Autodesk Fusion 360 part; units mm, degrees
(part 3 of 9)
  line L659 (-69.109, 106.2894) -> (-73.4391, 108.7894)
  line L660 (-63.2789, 108.7894) -> (-67.609, 106.2894)
  line L661 (-67.609, 106.2894) -> (-67.609, 101.2894)
  line L662 (-67.609, 101.2894) -> (-63.2789, 98.7894)
  line L663 (-63.2789, 98.7894) -> (-58.9487, 101.2894)
  line L664 (-58.9487, 101.2894) -> (-58.9487, 106.2894)
  line L665 (-58.9487, 106.2894) -> (-63.2789, 108.7894)
  line L666 (-53.1186, 108.7894) -> (-57.4487, 106.2894)
  line L667 (-57.4487, 106.2894) -> (-57.4487, 101.2894)
  line L668 (-57.4487, 101.2894) -> (-53.1186, 98.7894)
  line L669 (-53.1186, 98.7894) -> (-48.7885, 101.2894)
  line L670 (-48.7885, 101.2894) -> (-48.7885, 106.2894)
  line L671 (-48.7885, 106.2894) -> (-53.1186, 108.7894)
  line L672 (-42.9584, 108.7894) -> (-47.2885, 106.2894)
  line L673 (-47.2885, 106.2894) -> (-47.2885, 101.2894)
  line L674 (-47.2885, 101.2894) -> (-42.9584, 98.7894)
  line L675 (-42.9584, 98.7894) -> (-38.6282, 101.2894)
  line L676 (-38.6282, 101.2894) -> (-38.6282, 106.2894)
  line L677 (-38.6282, 106.2894) -> (-42.9584, 108.7894)
  line L678 (-32.7981, 108.7894) -> (-37.1282, 106.2894)
  line L679 (-37.1282, 106.2894) -> (-37.1282, 101.2894)
  line L680 (-37.1282, 101.2894) -> (-32.7981, 98.7894)
  line L681 (-32.7981, 98.7894) -> (-28.468, 101.2894)
  line L682 (-28.468, 101.2894) -> (-28.468, 106.2894)
  line L683 (-28.468, 106.2894) -> (-32.7981, 108.7894)
  line L684 (-22.6378, 108.7894) -> (-26.968, 106.2894)
  line L685 (-26.968, 106.2894) -> (-26.968, 101.2894)
  line L686 (-26.968, 101.2894) -> (-22.6378, 98.7894)
  line L687 (-22.6378, 98.7894) -> (-18.3077, 101.2894)
  line L688 (-18.3077, 101.2894) -> (-18.3077, 106.2894)
  line L689 (-18.3077, 106.2894) -> (-22.6378, 108.7894)
  line L690 (-12.4776, 108.7894) -> (-16.8077, 106.2894)
  line L691 (-16.8077, 106.2894) -> (-16.8077, 101.2894)
  line L692 (-16.8077, 101.2894) -> (-12.4776, 98.7894)
  line L693 (-12.4776, 98.7894) -> (-8.1475, 101.2894)
  line L694 (-8.1475, 101.2894) -> (-8.1475, 106.2894)
  line L695 (-8.1475, 106.2894) -> (-12.4776, 108.7894)
  line L696 (-109, 117.5885) -> (-113.3301, 115.0885)
  line L697 (-113.3301, 115.0885) -> (-113.3301, 110.0885)
  line L698 (-113.3301, 110.0885) -> (-109, 107.5885)
  line L699 (-109, 107.5885) -> (-104.6699, 110.0885)
  line L700 (-104.6699, 110.0885) -> (-104.6699, 115.0885)
  line L701 (-104.6699, 115.0885) -> (-109, 117.5885)
  line L702 (-98.8397, 117.5885) -> (-103.1699, 115.0885)
  line L703 (-103.1699, 115.0885) -> (-103.1699, 110.0885)
  line L704 (-103.1699, 110.0885) -> (-98.8397, 107.5885)
  line L705 (-98.8397, 107.5885) -> (-94.5096, 110.0885)
  line L706 (-94.5096, 110.0885) -> (-94.5096, 115.0885)
  line L707 (-94.5096, 115.0885) -> (-98.8397, 117.5885)
  line L708 (-88.6795, 117.5885) -> (-93.0096, 115.0885)
  line L709 (-93.0096, 115.0885) -> (-93.0096, 110.0885)
  line L710 (-93.0096, 110.0885) -> (-88.6795, 107.5885)
  line L711 (-88.6795, 107.5885) -> (-84.3494, 110.0885)
  line L712 (-84.3494, 110.0885) -> (-84.3494, 115.0885)
  line L713 (-84.3494, 115.0885) -> (-88.6795, 117.5885)
  line L714 (-78.5192, 117.5885) -> (-82.8494, 115.0885)
  line L715 (-82.8494, 115.0885) -> (-82.8494, 110.0885)
  line L716 (-82.8494, 110.0885) -> (-78.5192, 107.5885)
  line L717 (-78.5192, 107.5885) -> (-74.1891, 110.0885)
  line L718 (-74.1891, 110.0885) -> (-74.1891, 115.0885)
  line L719 (-74.1891, 115.0885) -> (-78.5192, 117.5885)
  line L720 (-68.359, 117.5885) -> (-72.6891, 115.0885)
  line L721 (-72.6891, 115.0885) -> (-72.6891, 110.0885)
  line L722 (-72.6891, 110.0885) -> (-68.359, 107.5885)
  line L723 (-68.359, 107.5885) -> (-64.0289, 110.0885)
  line L724 (-64.0289, 110.0885) -> (-64.0289, 115.0885)
  line L725 (-64.0289, 115.0885) -> (-68.359, 117.5885)
  line L726 (-58.1987, 117.5885) -> (-62.5289, 115.0885)
  line L727 (-62.5289, 115.0885) -> (-62.5289, 110.0885)
  line L728 (-62.5289, 110.0885) -> (-58.1987, 107.5885)
  line L729 (-58.1987, 107.5885) -> (-53.8686, 110.0885)
  line L730 (-53.8686, 110.0885) -> (-53.8686, 115.0885)
  line L731 (-53.8686, 115.0885) -> (-58.1987, 117.5885)
  line L732 (-48.0385, 117.5885) -> (-52.3686, 115.0885)
  line L733 (-52.3686, 115.0885) -> (-52.3686, 110.0885)
  line L734 (-52.3686, 110.0885) -> (-48.0385, 107.5885)
  line L735 (-48.0385, 107.5885) -> (-43.7084, 110.0885)
  line L736 (-43.7084, 110.0885) -> (-43.7084, 115.0885)
  line L737 (-43.7084, 115.0885) -> (-48.0385, 117.5885)
  line L738 (-37.8782, 117.5885) -> (-42.2084, 115.0885)
  line L739 (-42.2084, 115.0885) -> (-42.2084, 110.0885)
  line L740 (-42.2084, 110.0885) -> (-37.8782, 107.5885)
  line L741 (-37.8782, 107.5885) -> (-33.5481, 110.0885)
  line L742 (-33.5481, 110.0885) -> (-33.5481, 115.0885)
  line L743 (-33.5481, 115.0885) -> (-37.8782, 117.5885)
  line L744 (-27.718, 117.5885) -> (-32.0481, 115.0885)
  line L745 (-32.0481, 115.0885) -> (-32.0481, 110.0885)
  line L746 (-32.0481, 110.0885) -> (-27.718, 107.5885)
  line L747 (-27.718, 107.5885) -> (-23.3878, 110.0885)
  line L748 (-23.3878, 110.0885) -> (-23.3878, 115.0885)
  line L749 (-23.3878, 115.0885) -> (-27.718, 117.5885)
  line L750 (-17.5577, 117.5885) -> (-21.8878, 115.0885)
  line L751 (-21.8878, 115.0885) -> (-21.8878, 110.0885)
  line L752 (-21.8878, 110.0885) -> (-17.5577, 107.5885)
  line L753 (-17.5577, 107.5885) -> (-13.2276, 110.0885)
  line L754 (-13.2276, 110.0885) -> (-13.2276, 115.0885)
  line L755 (-13.2276, 115.0885) -> (-17.5577, 117.5885)
  line L756 (-7.3975, 117.5885) -> (-11.7276, 115.0885)
  line L757 (-11.7276, 115.0885) -> (-11.7276, 110.0885)
  line L758 (-11.7276, 110.0885) -> (-7.3975, 107.5885)
  line L759 (-7.3975, 107.5885) -> (-3.0673, 110.0885)
  line L760 (-3.0673, 110.0885) -> (-3.0673, 115.0885)
  line L761 (-3.0673, 115.0885) -> (-7.3975, 117.5885)
  line L762 (-103.9199, 126.3875) -> (-108.25, 123.8875)
  line L763 (-108.25, 123.8875) -> (-108.25, 118.8875)
  line L764 (-108.25, 118.8875) -> (-103.9199, 116.3875)
  line L765 (-103.9199, 116.3875) -> (-99.5897, 118.8875)
  line L766 (-99.5897, 118.8875) -> (-99.5897, 123.8875)
  line L767 (-99.5897, 123.8875) -> (-103.9199, 126.3875)
  line L768 (-93.7596, 126.3875) -> (-98.0897, 123.8875)
  line L769 (-98.0897, 123.8875) -> (-98.0897, 118.8875)
  line L770 (-98.0897, 118.8875) -> (-93.7596, 116.3875)
  line L771 (-93.7596, 116.3875) -> (-89.4295, 118.8875)
  line L772 (-89.4295, 118.8875) -> (-89.4295, 123.8875)
  line L773 (-89.4295, 123.8875) -> (-93.7596, 126.3875)
  line L774 (-83.5994, 126.3875) -> (-87.9295, 123.8875)
  line L775 (-87.9295, 123.8875) -> (-87.9295, 118.8875)
  line L776 (-87.9295, 118.8875) -> (-83.5994, 116.3875)
  line L777 (-83.5994, 116.3875) -> (-79.2692, 118.8875)
  line L778 (-79.2692, 118.8875) -> (-79.2692, 123.8875)
  line L779 (-79.2692, 123.8875) -> (-83.5994, 126.3875)
  line L780 (-73.4391, 126.3875) -> (-77.7692, 123.8875)
  line L781 (-77.7692, 123.8875) -> (-77.7692, 118.8875)
  line L782 (-77.7692, 118.8875) -> (-73.4391, 116.3875)
  line L783 (-73.4391, 116.3875) -> (-69.109, 118.8875)
  line L784 (-69.109, 118.8875) -> (-69.109, 123.8875)
  line L785 (-69.109, 123.8875) -> (-73.4391, 126.3875)
  line L786 (-63.2789, 126.3875) -> (-67.609, 123.8875)
  line L787 (-67.609, 123.8875) -> (-67.609, 118.8875)
  line L788 (-67.609, 118.8875) -> (-63.2789, 116.3875)
  line L789 (-63.2789, 116.3875) -> (-58.9487, 118.8875)
  line L790 (-58.9487, 118.8875) -> (-58.9487, 123.8875)
  line L791 (-58.9487, 123.8875) -> (-63.2789, 126.3875)
  line L792 (-53.1186, 126.3875) -> (-57.4487, 123.8875)
  line L793 (-57.4487, 123.8875) -> (-57.4487, 118.8875)
  line L794 (-57.4487, 118.8875) -> (-53.1186, 116.3875)
  line L795 (-53.1186, 116.3875) -> (-48.7885, 118.8875)
  line L796 (-48.7885, 118.8875) -> (-48.7885, 123.8875)
  line L797 (-48.7885, 123.8875) -> (-53.1186, 126.3875)
  line L798 (-42.9584, 126.3875) -> (-47.2885, 123.8875)
  line L799 (-47.2885, 123.8875) -> (-47.2885, 118.8875)
  line L800 (-47.2885, 118.8875) -> (-42.9584, 116.3875)
  line L801 (-42.9584, 116.3875) -> (-38.6282, 118.8875)
  line L802 (-38.6282, 118.8875) -> (-38.6282, 123.8875)
  line L803 (-38.6282, 123.8875) -> (-42.9584, 126.3875)
  line L804 (-32.7981, 126.3875) -> (-37.1282, 123.8875)
  line L805 (-37.1282, 123.8875) -> (-37.1282, 118.8875)
  line L806 (-37.1282, 118.8875) -> (-32.7981, 116.3875)
  line L807 (-32.7981, 116.3875) -> (-28.468, 118.8875)
  line L808 (-28.468, 118.8875) -> (-28.468, 123.8875)
  line L809 (-28.468, 123.8875) -> (-32.7981, 126.3875)
  line L810 (-22.6378, 126.3875) -> (-26.968, 123.8875)
  line L811 (-26.968, 123.8875) -> (-26.968, 118.8875)
  line L812 (-26.968, 118.8875) -> (-22.6378, 116.3875)
  line L813 (-22.6378, 116.3875) -> (-18.3077, 118.8875)
  line L814 (-18.3077, 118.8875) -> (-18.3077, 123.8875)
  line L815 (-18.3077, 123.8875) -> (-22.6378, 126.3875)
  line L816 (-12.4776, 126.3875) -> (-16.8077, 123.8875)
  line L817 (-16.8077, 123.8875) -> (-16.8077, 118.8875)
  line L818 (-16.8077, 118.8875) -> (-12.4776, 116.3875)
  line L819 (-12.4776, 116.3875) -> (-8.1475, 118.8875)
  line L820 (-8.1475, 118.8875) -> (-8.1475, 123.8875)
  line L821 (-8.1475, 123.8875) -> (-12.4776, 126.3875)
  line L822 (-109, 135.1865) -> (-113.3301, 132.6865)
  line L823 (-113.3301, 132.6865) -> (-113.3301, 127.6865)
  line L824 (-113.3301, 127.6865) -> (-109, 125.1865)
  line L825 (-109, 125.1865) -> (-104.6699, 127.6865)
  line L826 (-104.6699, 127.6865) -> (-104.6699, 132.6865)
  line L827 (-104.6699, 132.6865) -> (-109, 135.1865)
  line L828 (-98.8397, 135.1865) -> (-103.1699, 132.6865)
  line L829 (-103.1699, 132.6865) -> (-103.1699, 127.6865)
  line L830 (-103.1699, 127.6865) -> (-98.8397, 125.1865)
  line L831 (-98.8397, 125.1865) -> (-94.5096, 127.6865)
  line L832 (-94.5096, 127.6865) -> (-94.5096, 132.6865)
  line L833 (-94.5096, 132.6865) -> (-98.8397, 135.1865)
  line L834 (-88.6795, 135.1865) -> (-93.0096, 132.6865)
  line L835 (-93.0096, 132.6865) -> (-93.0096, 127.6865)
  line L836 (-93.0096, 127.6865) -> (-88.6795, 125.1865)
  line L837 (-88.6795, 125.1865) -> (-84.3494, 127.6865)
  line L838 (-84.3494, 127.6865) -> (-84.3494, 132.6865)
  line L839 (-84.3494, 132.6865) -> (-88.6795, 135.1865)
  line L840 (-78.5192, 135.1865) -> (-82.8494, 132.6865)
  line L841 (-82.8494, 132.6865) -> (-82.8494, 127.6865)
  line L842 (-82.8494, 127.6865) -> (-78.5192, 125.1865)
  line L843 (-78.5192, 125.1865) -> (-74.1891, 127.6865)
  line L844 (-74.1891, 127.6865) -> (-74.1891, 132.6865)
  line L845 (-74.1891, 132.6865) -> (-78.5192, 135.1865)
  line L846 (-68.359, 135.1865) -> (-72.6891, 132.6865)
  line L847 (-72.6891, 132.6865) -> (-72.6891, 127.6865)
  line L848 (-72.6891, 127.6865) -> (-68.359, 125.1865)
  line L849 (-68.359, 125.1865) -> (-64.0289, 127.6865)
  line L850 (-64.0289, 127.6865) -> (-64.0289, 132.6865)
  line L851 (-64.0289, 132.6865) -> (-68.359, 135.1865)
  line L852 (-58.1987, 135.1865) -> (-62.5289, 132.6865)
  line L853 (-62.5289, 132.6865) -> (-62.5289, 127.6865)
  line L854 (-62.5289, 127.6865) -> (-58.1987, 125.1865)
  line L855 (-58.1987, 125.1865) -> (-53.8686, 127.6865)
  line L856 (-53.8686, 127.6865) -> (-53.8686, 132.6865)
  line L857 (-53.8686, 132.6865) -> (-58.1987, 135.1865)
  line L858 (-48.0385, 135.1865) -> (-52.3686, 132.6865)
  line L859 (-52.3686, 132.6865) -> (-52.3686, 127.6865)
  line L860 (-52.3686, 127.6865) -> (-48.0385, 125.1865)
  line L861 (-48.0385, 125.1865) -> (-43.7084, 127.6865)
  line L862 (-43.7084, 127.6865) -> (-43.7084, 132.6865)
  line L863 (-43.7084, 132.6865) -> (-48.0385, 135.1865)
  line L864 (-37.8782, 135.1865) -> (-42.2084, 132.6865)
  line L865 (-42.2084, 132.6865) -> (-42.2084, 127.6865)
  line L866 (-42.2084, 127.6865) -> (-37.8782, 125.1865)
  line L867 (-37.8782, 125.1865) -> (-33.5481, 127.6865)
  line L868 (-33.5481, 127.6865) -> (-33.5481, 132.6865)
  line L869 (-33.5481, 132.6865) -> (-37.8782, 135.1865)
  line L870 (-27.718, 135.1865) -> (-32.0481, 132.6865)
  line L871 (-32.0481, 132.6865) -> (-32.0481, 127.6865)
  line L872 (-32.0481, 127.6865) -> (-27.718, 125.1865)
  line L873 (-27.718, 125.1865) -> (-23.3878, 127.6865)
  line L874 (-23.3878, 127.6865) -> (-23.3878, 132.6865)
  line L875 (-23.3878, 132.6865) -> (-27.718, 135.1865)
  line L876 (-17.5577, 135.1865) -> (-21.8878, 132.6865)
  line L877 (-21.8878, 132.6865) -> (-21.8878, 127.6865)
  line L878 (-21.8878, 127.6865) -> (-17.5577, 125.1865)
  line L879 (-17.5577, 125.1865) -> (-13.2276, 127.6865)
  line L880 (-13.2276, 127.6865) -> (-13.2276, 132.6865)
  line L881 (-13.2276, 132.6865) -> (-17.5577, 135.1865)
  line L882 (-7.3975, 135.1865) -> (-11.7276, 132.6865)
  line L883 (-11.7276, 132.6865) -> (-11.7276, 127.6865)
  line L884 (-11.7276, 127.6865) -> (-7.3975, 125.1865)
  line L885 (-7.3975, 125.1865) -> (-3.0673, 127.6865)
  line L886 (-3.0673, 127.6865) -> (-3.0673, 132.6865)
  line L887 (-3.0673, 132.6865) -> (-7.3975, 135.1865)
  line L888 (-103.9199, 143.9856) -> (-108.25, 141.4856)
  line L889 (-108.25, 141.4856) -> (-108.25, 136.4856)
  line L890 (-108.25, 136.4856) -> (-103.9199, 133.9856)
  line L891 (-103.9199, 133.9856) -> (-99.5897, 136.4856)
  line L892 (-99.5897, 136.4856) -> (-99.5897, 141.4856)
  line L893 (-99.5897, 141.4856) -> (-103.9199, 143.9856)
  line L894 (-93.7596, 143.9856) -> (-98.0897, 141.4856)
  line L895 (-98.0897, 141.4856) -> (-98.0897, 136.4856)
  line L896 (-98.0897, 136.4856) -> (-93.7596, 133.9856)
  line L897 (-93.7596, 133.9856) -> (-89.4295, 136.4856)
  line L898 (-89.4295, 136.4856) -> (-89.4295, 141.4856)
  line L899 (-89.4295, 141.4856) -> (-93.7596, 143.9856)
  line L900 (-83.5994, 143.9856) -> (-87.9295, 141.4856)
  line L901 (-87.9295, 141.4856) -> (-87.9295, 136.4856)
  line L902 (-87.9295, 136.4856) -> (-83.5994, 133.9856)
  line L903 (-83.5994, 133.9856) -> (-79.2692, 136.4856)
  line L904 (-79.2692, 136.4856) -> (-79.2692, 141.4856)
  line L905 (-79.2692, 141.4856) -> (-83.5994, 143.9856)
  line L906 (-73.4391, 143.9856) -> (-77.7692, 141.4856)
  line L907 (-77.7692, 141.4856) -> (-77.7692, 136.4856)
  line L908 (-77.7692, 136.4856) -> (-73.4391, 133.9856)
  line L909 (-73.4391, 133.9856) -> (-69.109, 136.4856)
  line L910 (-69.109, 136.4856) -> (-69.109, 141.4856)
  line L911 (-69.109, 141.4856) -> (-73.4391, 143.9856)
  line L912 (-63.2789, 143.9856) -> (-67.609, 141.4856)
  line L913 (-67.609, 141.4856) -> (-67.609, 136.4856)
  line L914 (-67.609, 136.4856) -> (-63.2789, 133.9856)
  line L915 (-63.2789, 133.9856) -> (-58.9487, 136.4856)
  line L916 (-58.9487, 136.4856) -> (-58.9487, 141.4856)
  line L917 (-58.9487, 141.4856) -> (-63.2789, 143.9856)
  line L918 (-53.1186, 143.9856) -> (-57.4487, 141.4856)
  line L919 (-57.4487, 141.4856) -> (-57.4487, 136.4856)
  line L920 (-57.4487, 136.4856) -> (-53.1186, 133.9856)
  line L921 (-53.1186, 133.9856) -> (-48.7885, 136.4856)
  line L922 (-48.7885, 136.4856) -> (-48.7885, 141.4856)
  line L923 (-48.7885, 141.4856) -> (-53.1186, 143.9856)
  line L924 (-42.9584, 143.9856) -> (-47.2885, 141.4856)
  line L925 (-47.2885, 141.4856) -> (-47.2885, 136.4856)
  line L926 (-47.2885, 136.4856) -> (-42.9584, 133.9856)
  line L927 (-42.9584, 133.9856) -> (-38.6282, 136.4856)
  line L928 (-38.6282, 136.4856) -> (-38.6282, 141.4856)
  line L929 (-38.6282, 141.4856) -> (-42.9584, 143.9856)
  line L930 (-32.7981, 143.9856) -> (-37.1282, 141.4856)
  line L931 (-37.1282, 141.4856) -> (-37.1282, 136.4856)
  line L932 (-37.1282, 136.4856) -> (-32.7981, 133.9856)
  line L933 (-32.7981, 133.9856) -> (-28.468, 136.4856)
  line L934 (-28.468, 136.4856) -> (-28.468, 141.4856)
  line L935 (-28.468, 141.4856) -> (-32.7981, 143.9856)
  line L936 (-22.6378, 143.9856) -> (-26.968, 141.4856)
  line L937 (-26.968, 141.4856) -> (-26.968, 136.4856)
  line L938 (-26.968, 136.4856) -> (-22.6378, 133.9856)
  line L939 (-22.6378, 133.9856) -> (-18.3077, 136.4856)
  line L940 (-18.3077, 136.4856) -> (-18.3077, 141.4856)
  line L941 (-18.3077, 141.4856) -> (-22.6378, 143.9856)
  line L942 (-12.4776, 143.9856) -> (-16.8077, 141.4856)
  line L943 (-16.8077, 141.4856) -> (-16.8077, 136.4856)
  line L944 (-16.8077, 136.4856) -> (-12.4776, 133.9856)
  line L945 (-12.4776, 133.9856) -> (-8.1475, 136.4856)
  line L946 (-8.1475, 136.4856) -> (-8.1475, 141.4856)
  line L947 (-8.1475, 141.4856) -> (-12.4776, 143.9856)
  line L948 (-109, 152.7846) -> (-113.3301, 150.2846)
  line L949 (-113.3301, 150.2846) -> (-113.3301, 145.2846)
  line L950 (-113.3301, 145.2846) -> (-109, 142.7846)
  line L951 (-109, 142.7846) -> (-104.6699, 145.2846)
  line L952 (-104.6699, 145.2846) -> (-104.6699, 150.2846)
  line L953 (-104.6699, 150.2846) -> (-109, 152.7846)
  line L954 (-98.8397, 152.7846) -> (-103.1699, 150.2846)
  line L955 (-103.1699, 150.2846) -> (-103.1699, 145.2846)
  line L956 (-103.1699, 145.2846) -> (-98.8397, 142.7846)
  line L957 (-98.8397, 142.7846) -> (-94.5096, 145.2846)
  line L958 (-94.5096, 145.2846) -> (-94.5096, 150.2846)
  line L959 (-94.5096, 150.2846) -> (-98.8397, 152.7846)
  line L960 (-88.6795, 152.7846) -> (-93.0096, 150.2846)
  line L961 (-93.0096, 150.2846) -> (-93.0096, 145.2846)
  line L962 (-93.0096, 145.2846) -> (-88.6795, 142.7846)
  line L963 (-88.6795, 142.7846) -> (-84.3494, 145.2846)
  line L964 (-84.3494, 145.2846) -> (-84.3494, 150.2846)
  line L965 (-84.3494, 150.2846) -> (-88.6795, 152.7846)
  line L966 (-78.5192, 152.7846) -> (-82.8494, 150.2846)
  line L967 (-82.8494, 150.2846) -> (-82.8494, 145.2846)
  line L968 (-82.8494, 145.2846) -> (-78.5192, 142.7846)
  line L969 (-78.5192, 142.7846) -> (-74.1891, 145.2846)
  line L970 (-74.1891, 145.2846) -> (-74.1891, 150.2846)
  line L971 (-74.1891, 150.2846) -> (-78.5192, 152.7846)
  line L972 (-68.359, 152.7846) -> (-72.6891, 150.2846)
  line L973 (-72.6891, 150.2846) -> (-72.6891, 145.2846)
  line L974 (-72.6891, 145.2846) -> (-68.359, 142.7846)
  line L975 (-68.359, 142.7846) -> (-64.0289, 145.2846)
  line L976 (-64.0289, 145.2846) -> (-64.0289, 150.2846)
  line L977 (-64.0289, 150.2846) -> (-68.359, 152.7846)
  line L978 (-58.1987, 152.7846) -> (-62.5289, 150.2846)
  line L979 (-62.5289, 150.2846) -> (-62.5289, 145.2846)
  line L980 (-62.5289, 145.2846) -> (-58.1987, 142.7846)
  line L981 (-58.1987, 142.7846) -> (-53.8686, 145.2846)
  line L982 (-53.8686, 145.2846) -> (-53.8686, 150.2846)
  line L983 (-53.8686, 150.2846) -> (-58.1987, 152.7846)
  line L984 (-48.0385, 152.7846) -> (-52.3686, 150.2846)
  line L985 (-52.3686, 150.2846) -> (-52.3686, 145.2846)
  line L986 (-52.3686, 145.2846) -> (-48.0385, 142.7846)
  line L987 (-48.0385, 142.7846) -> (-43.7084, 145.2846)
  line L988 (-43.7084, 145.2846) -> (-43.7084, 150.2846)
  line L989 (-43.7084, 150.2846) -> (-48.0385, 152.7846)
  line L990 (-37.8782, 152.7846) -> (-42.2084, 150.2846)
  line L991 (-42.2084, 150.2846) -> (-42.2084, 145.2846)
  line L992 (-42.2084, 145.2846) -> (-37.8782, 142.7846)
  line L993 (-37.8782, 142.7846) -> (-33.5481, 145.2846)
  line L994 (-33.5481, 145.2846) -> (-33.5481, 150.2846)
  line L995 (-33.5481, 150.2846) -> (-37.8782, 152.7846)
  line L996 (-27.718, 152.7846) -> (-32.0481, 150.2846)
  line L997 (-32.0481, 150.2846) -> (-32.0481, 145.2846)
  line L998 (-32.0481, 145.2846) -> (-27.718, 142.7846)
  line L999 (-27.718, 142.7846) -> (-23.3878, 145.2846)
  line L1000 (-23.3878, 145.2846) -> (-23.3878, 150.2846)
  line L1001 (-23.3878, 150.2846) -> (-27.718, 152.7846)
  line L1002 (-17.5577, 152.7846) -> (-21.8878, 150.2846)
  line L1003 (-21.8878, 150.2846) -> (-21.8878, 145.2846)
  line L1004 (-21.8878, 145.2846) -> (-17.5577, 142.7846)
  line L1005 (-17.5577, 142.7846) -> (-13.2276, 145.2846)
  line L1006 (-13.2276, 145.2846) -> (-13.2276, 150.2846)
  line L1007 (-13.2276, 150.2846) -> (-17.5577, 152.7846)
  line L1008 (-7.3975, 152.7846) -> (-11.7276, 150.2846)
  line L1009 (-11.7276, 150.2846) -> (-11.7276, 145.2846)
  line L1010 (-11.7276, 145.2846) -> (-7.3975, 142.7846)
  line L1011 (-7.3975, 142.7846) -> (-3.0673, 145.2846)
  line L1012 (-3.0673, 145.2846) -> (-3.0673, 150.2846)
  line L1013 (-3.0673, 150.2846) -> (-7.3975, 152.7846)
extrude "拉伸22" cut sketch "草图21" against normal blind 5 contours L6 L7 L8 L9 L10 L11 | L12 L13 L14 L15 L16 L17 | L18 L19 L20 L21 L22 L23 | L24 L25 L26 L27 L28 L29 | L30 L31 L32 L33 L34 L35 | L36 L37 L38 L39 L40 L41 | L42 L43 L44 L45 L46 L47 | L48 L49 L50 L51 L52 L53 | L54 L55 L56 L57 L58 L59 | L60 L61 L62 L63 L64 L65 | L66 L67 L68 L69 L70 L71 | L72 L73 L74 L75 L76 L77 | L78 L79 L80 L81 L82 L83 | L84 L85 L86 L87 L88 L89 | L90 L91 L92 L93 L94 L95 | L96 L97 L98 L99 L100 L101 | L102 L103 L104 L105 L106 L107 | L108 L109 L110 L111 L112 L113 | L114 L115 L116 L117 L118 L119 | L120 L121 L122 L123 L124 L125 | L126 L127 L128 L129 L130 L131 | L132 L133 L134 L135 L136 L137 | L138 L139 L140 L141 L142 L143 | L144 L145 L146 L147 L148 L149 | L150 L151 L152 L153 L154 L155 | L156 L157 L158 L159 L160 L161 | L162 L163 L164 L165 L166 L167 | L168 L169 L170 L171 L172 L173 | L174 L175 L176 L177 L178 L179 | L180 L181 L182 L183 L184 L185 | L186 L187 L188 L189 L190 L191 | L192 L193 L194 L195 L196 L197 | L198 L199 L200 L201 L202 L203 | L204 L205 L206 L207 L208 L209 | L210 L211 L212 L213 L214 L215 | L216 L217 L218 L219 L220 L221 | L222 L223 L224 L225 L226 L227 | L228 L229 L230 L231 L232 L233 | L234 L235 L236 L237 L238 L239 | L240 L241 L242 L243 L244 L245 | L246 L247 L248 L249 L250 L251 | L252 L253 L254 L255 L256 L257 | L258 L259 L260 L261 L262 L263 | L264 L265 L266 L267 L268 L269 | L270 L271 L272 L273 L274 L275 | L276 L277 L278 L279 L280 L281 | L282 L283 L284 L285 L286 L287 | L288 L289 L290 L291 L292 L293 | L294 L295 L296 L297 L298 L299 | L300 L301 L302 L303 L304 L305 | L306 L307 L308 L309 L310 L311 | L312 L313 L314 L315 L316 L317 | L318 L319 L320 L321 L322 L323 | L324 L325 L326 L327 L328 L329 | L330 L331 L332 L333 L334 L335 | L336 L337 L338 L339 L340 L341 | L342 L343 L344 L345 L346 L347 | L348 L349 L350 L351 L352 L353 | L354 L355 L356 L357 L358 L359 | L360 L361 L362 L363 L364 L365 | L366 L367 L368 L369 L370 L371 | L372 L373 L374 L375 L376 L377 | L378 L379 L380 L381 L382 L383 | L384 L385 L386 L387 L388 L389 | L390 L391 L392 L393 L394 L395 | L396 L397 L398 L399 L400 L401 | L402 L403 L404 L405 L406 L407 | L408 L409 L410 L411 L412 L413 | L414 L415 L416 L417 L418 L419 | L420 L421 L422 L423 L424 L425 | L426 L427 L428 L429 L430 L431 | L432 L433 L434 L435 L436 L437 | L438 L439 L440 L441 L442 L443 | L444 L445 L446 L447 L448 L449 | L450 L451 L452 L453 L454 L455 | L456 L457 L458 L459 L460 L461 | L462 L463 L464 L465 L466 L467 | L468 L469 L470 L471 L472 L473 | L474 L475 L476 L477 L478 L479 | L480 L481 L482 L483 L484 L485 | L486 L487 L488 L489 L490 L491 | L492 L493 L494 L495 L496 L497 | L498 L499 L500 L501 L502 L503 | L504 L505 L506 L507 L508 L509 | L510 L511 L512 L513 L514 L515 | L516 L517 L518 L519 L520 L521 | L522 L523 L524 L525 L526 L527 | L528 L529 L530 L531 L532 L533 | L534 L535 L536 L537 L538 L539 | L540 L541 L542 L543 L544 L545 | L546 L547 L548 L549 L550 L551 | L552 L553 L554 L555 L556 L557 | L558 L559 L560 L561 L562 L563 | L564 L565 L566 L567 L568 L569 | L570 L571 L572 L573 L574 L575 | L576 L577 L578 L579 L580 L581 | L582 L583 L584 L585 L586 L587 | L588 L589 L590 L591 L592 L593 | L594 L595 L596 L597 L598 L599 | L600 L601 L602 L603 L604 L605 | L606 L607 L608 L609 L610 L611 | L612 L613 L614 L615 L616 L617 | L618 L619 L620 L621 L622 L623 | L624 L625 L626 L627 L628 L629 | L630 L631 L632 L633 L634 L635 | L636 L637 L638 L639 L640 L641 | L642 L643 L644 L645 L646 L647 | L648 L649 L650 L651 L652 L653 | L654 L655 L656 L657 L658 L659 | L660 L661 L662 L663 L664 L665 | L666 L667 L668 L669 L670 L671 | L672 L673 L674 L675 L676 L677 | L678 L679 L680 L681 L682 L683 | L684 L685 L686 L687 L688 L689 | L690 L691 L692 L693 L694 L695 | L696 L697 L698 L699 L700 L701 | L702 L703 L704 L705 L706 L707 | L708 L709 L710 L711 L712 L713 | L714 L715 L716 L717 L718 L719 | L720 L721 L722 L723 L724 L725 | L726 L727 L728 L729 L730 L731 | L732 L733 L734 L735 L736 L737 | L738 L739 L740 L741 L742 L743 | L744 L745 L746 L747 L748 L749 | L750 L751 L752 L753 L754 L755 | L756 L757 L758 L759 L760 L761 | L762 L763 L764 L765 L766 L767 | L768 L769 L770 L771 L772 L773 | L774 L775 L776 L777 L778 L779 | L780 L781 L782 L783 L784 L785 | L786 L787 L788 L789 L790 L791 | L792 L793 L794 L795 L796 L797 | L798 L799 L800 L801 L802 L803 | L804 L805 L806 L807 L808 L809 | L810 L811 L812 L813 L814 L815 | L816 L817 L818 L819 L820 L821 | L822 L823 L824 L825 L826 L827 | L828 L829 L830 L831 L832 L833 | L834 L835 L836 L837 L838 L839 | L840 L841 L842 L843 L844 L845 | L846 L847 L848 L849 L850 L851 | L852 L853 L854 L855 L856 L857 | L858 L859 L860 L861 L862 L863 | L864 L865 L866 L867 L868 L869 | L870 L871 L872 L873 L874 L875 | L876 L877 L878 L879 L880 L881 | L882 L883 L884 L885 L886 L887 | L888 L889 L890 L891 L892 L893 | L894 L895 L896 L897 L898 L899 | L900 L901 L902 L903 L904 L905 | L906 L907 L908 L909 L910 L911 | L912 L913 L914 L915 L916 L917 | L918 L919 L920 L921 L922 L923 | L924 L925 L926 L927 L928 L929 | L930 L931 L932 L933 L934 L935 | L936 L937 L938 L939 L940 L941 | L942 L943 L944 L945 L946 L947 | L948 L949 L950 L951 L952 L953 | L954 L955 L956 L957 L958 L959 | L960 L961 L962 L963 L964 L965 | L966 L967 L968 L969 L970 L971 | L972 L973 L974 L975 L976 L977 | L978 L979 L980 L981 L982 L983 | L984 L985 L986 L987 L988 L989 | L990 L991 L992 L993 L994 L995 | L996 L997 L998 L999 L1000 L1001 | L1002 L1003 L1004 L1005 L1006 L1007 | L1008 L1009 L1010 L1011 L1012 L1013 bodies 1
sketch "草图22" plane through (-116, 0, 0) normal (1, 0, 0) x (0, 1, 0)
  line L0 (-4, 65) -> (-3.998, 65)
  line L1 (-3.998, 65) -> (-3.998, 0)
  line L2 (-3.998, 0) -> (116, 0)
  line L3 (116, 0) -> (116, 160)
  line L4 (116, 160) -> (-4, 160)
  line L5 (-4, 160) -> (-4, 65)
  line L6 (8.0801, 20.799) -> (3.75, 18.299)
  line L7 (3.75, 18.299) -> (3.75, 13.299)
  line L8 (3.75, 13.299) -> (8.0801, 10.799)
  line L9 (8.0801, 10.799) -> (12.4103, 13.299)
  line L10 (12.4103, 13.299) -> (12.4103, 18.299)
  line L11 (12.4103, 18.299) -> (8.0801, 20.799)
  line L12 (18.2404, 20.799) -> (13.9103, 18.299)
  line L13 (13.9103, 18.299) -> (13.9103, 13.299)
  line L14 (13.9103, 13.299) -> (18.2404, 10.799)
  line L15 (18.2404, 10.799) -> (22.5705, 13.299)
  line L16 (22.5705, 13.299) -> (22.5705, 18.299)
  line L17 (22.5705, 18.299) -> (18.2404, 20.799)
  line L18 (28.4006, 20.799) -> (24.0705, 18.299)
  line L19 (24.0705, 18.299) -> (24.0705, 13.299)
  line L20 (24.0705, 13.299) -> (28.4006, 10.799)
  line L21 (28.4006, 10.799) -> (32.7308, 13.299)
  line L22 (32.7308, 13.299) -> (32.7308, 18.299)
  line L23 (32.7308, 18.299) -> (28.4006, 20.799)
  line L24 (38.5609, 20.799) -> (34.2308, 18.299)
  line L25 (34.2308, 18.299) -> (34.2308, 13.299)
  line L26 (34.2308, 13.299) -> (38.5609, 10.799)
  line L27 (38.5609, 10.799) -> (42.891, 13.299)
  line L28 (42.891, 13.299) -> (42.891, 18.299)
  line L29 (42.891, 18.299) -> (38.5609, 20.799)
  line L30 (48.7211, 20.799) -> (44.391, 18.299)
  line L31 (44.391, 18.299) -> (44.391, 13.299)
  line L32 (44.391, 13.299) -> (48.7211, 10.799)
  line L33 (48.7211, 10.799) -> (53.0513, 13.299)
  line L34 (53.0513, 13.299) -> (53.0513, 18.299)
  line L35 (53.0513, 18.299) -> (48.7211, 20.799)
  line L36 (58.8814, 20.799) -> (54.5513, 18.299)
  line L37 (54.5513, 18.299) -> (54.5513, 13.299)
  line L38 (54.5513, 13.299) -> (58.8814, 10.799)
  line L39 (58.8814, 10.799) -> (63.2115, 13.299)
  line L40 (63.2115, 13.299) -> (63.2115, 18.299)
  line L41 (63.2115, 18.299) -> (58.8814, 20.799)
  line L42 (69.0417, 20.799) -> (64.7115, 18.299)
  line L43 (64.7115, 18.299) -> (64.7115, 13.299)
  line L44 (64.7115, 13.299) -> (69.0417, 10.799)
  line L45 (69.0417, 10.799) -> (73.3718, 13.299)
  line L46 (73.3718, 13.299) -> (73.3718, 18.299)
  line L47 (73.3718, 18.299) -> (69.0417, 20.799)
  line L48 (79.2019, 20.799) -> (74.8718, 18.299)
  line L49 (74.8718, 18.299) -> (74.8718, 13.299)
  line L50 (74.8718, 13.299) -> (79.2019, 10.799)
  line L51 (79.2019, 10.799) -> (83.532, 13.299)
  line L52 (83.532, 13.299) -> (83.532, 18.299)
  line L53 (83.532, 18.299) -> (79.2019, 20.799)
  line L54 (89.3622, 20.799) -> (85.032, 18.299)
  line L55 (85.032, 18.299) -> (85.032, 13.299)
  line L56 (85.032, 13.299) -> (89.3622, 10.799)
  line L57 (89.3622, 10.799) -> (93.6923, 13.299)
  line L58 (93.6923, 13.299) -> (93.6923, 18.299)
  line L59 (93.6923, 18.299) -> (89.3622, 20.799)
  line L60 (99.5224, 20.799) -> (95.1923, 18.299)
  line L61 (95.1923, 18.299) -> (95.1923, 13.299)
  line L62 (95.1923, 13.299) -> (99.5224, 10.799)
  line L63 (99.5224, 10.799) -> (103.8525, 13.299)
  line L64 (103.8525, 13.299) -> (103.8525, 18.299)
  line L65 (103.8525, 18.299) -> (99.5224, 20.799)
  line L66 (3, 29.5981) -> (-1.3301, 27.0981)
  line L67 (-1.3301, 27.0981) -> (-1.3301, 22.0981)
  line L68 (-1.3301, 22.0981) -> (3, 19.5981)
  line L69 (3, 19.5981) -> (7.3301, 22.0981)
  line L70 (7.3301, 22.0981) -> (7.3301, 27.0981)
  line L71 (7.3301, 27.0981) -> (3, 29.5981)
  line L72 (13.1603, 29.5981) -> (8.8301, 27.0981)
  line L73 (8.8301, 27.0981) -> (8.8301, 22.0981)
  line L74 (8.8301, 22.0981) -> (13.1603, 19.5981)
  line L75 (13.1603, 19.5981) -> (17.4904, 22.0981)
  line L76 (17.4904, 22.0981) -> (17.4904, 27.0981)
  line L77 (17.4904, 27.0981) -> (13.1603, 29.5981)
  line L78 (23.3205, 29.5981) -> (18.9904, 27.0981)
  line L79 (18.9904, 27.0981) -> (18.9904, 22.0981)
  line L80 (18.9904, 22.0981) -> (23.3205, 19.5981)
  line L81 (23.3205, 19.5981) -> (27.6506, 22.0981)
  line L82 (27.6506, 22.0981) -> (27.6506, 27.0981)
  line L83 (27.6506, 27.0981) -> (23.3205, 29.5981)
  line L84 (33.4808, 29.5981) -> (29.1506, 27.0981)
  line L85 (29.1506, 27.0981) -> (29.1506, 22.0981)
  line L86 (29.1506, 22.0981) -> (33.4808, 19.5981)
  line L87 (33.4808, 19.5981) -> (37.8109, 22.0981)
  line L88 (37.8109, 22.0981) -> (37.8109, 27.0981)
  line L89 (37.8109, 27.0981) -> (33.4808, 29.5981)
  line L90 (43.641, 29.5981) -> (39.3109, 27.0981)
  line L91 (39.3109, 27.0981) -> (39.3109, 22.0981)
  line L92 (39.3109, 22.0981) -> (43.641, 19.5981)
  line L93 (43.641, 19.5981) -> (47.9711, 22.0981)
  line L94 (47.9711, 22.0981) -> (47.9711, 27.0981)
  line L95 (47.9711, 27.0981) -> (43.641, 29.5981)
  line L96 (53.8013, 29.5981) -> (49.4711, 27.0981)
  line L97 (49.4711, 27.0981) -> (49.4711, 22.0981)
  line L98 (49.4711, 22.0981) -> (53.8013, 19.5981)
  line L99 (53.8013, 19.5981) -> (58.1314, 22.0981)
  line L100 (58.1314, 22.0981) -> (58.1314, 27.0981)
  line L101 (58.1314, 27.0981) -> (53.8013, 29.5981)
  line L102 (63.9615, 29.5981) -> (59.6314, 27.0981)
  line L103 (59.6314, 27.0981) -> (59.6314, 22.0981)
  line L104 (59.6314, 22.0981) -> (63.9615, 19.5981)
  line L105 (63.9615, 19.5981) -> (68.2917, 22.0981)
  line L106 (68.2917, 22.0981) -> (68.2917, 27.0981)
  line L107 (68.2917, 27.0981) -> (63.9615, 29.5981)
  line L108 (74.1218, 29.5981) -> (69.7917, 27.0981)
  line L109 (69.7917, 27.0981) -> (69.7917, 22.0981)
  line L110 (69.7917, 22.0981) -> (74.1218, 19.5981)
  line L111 (74.1218, 19.5981) -> (78.4519, 22.0981)
  line L112 (78.4519, 22.0981) -> (78.4519, 27.0981)
  line L113 (78.4519, 27.0981) -> (74.1218, 29.5981)
  line L114 (84.282, 29.5981) -> (79.9519, 27.0981)
  line L115 (79.9519, 27.0981) -> (79.9519, 22.0981)
  line L116 (79.9519, 22.0981) -> (84.282, 19.5981)
  line L117 (84.282, 19.5981) -> (88.6122, 22.0981)
  line L118 (88.6122, 22.0981) -> (88.6122, 27.0981)
  line L119 (88.6122, 27.0981) -> (84.282, 29.5981)
  line L120 (94.4423, 29.5981) -> (90.1122, 27.0981)
  line L121 (90.1122, 27.0981) -> (90.1122, 22.0981)
  line L122 (90.1122, 22.0981) -> (94.4423, 19.5981)
  line L123 (94.4423, 19.5981) -> (98.7724, 22.0981)
  line L124 (98.7724, 22.0981) -> (98.7724, 27.0981)
  line L125 (98.7724, 27.0981) -> (94.4423, 29.5981)
  line L126 (104.6025, 29.5981) -> (100.2724, 27.0981)
  line L127 (100.2724, 27.0981) -> (100.2724, 22.0981)
  line L128 (100.2724, 22.0981) -> (104.6025, 19.5981)
  line L129 (104.6025, 19.5981) -> (108.9327, 22.0981)
  line L130 (108.9327, 22.0981) -> (108.9327, 27.0981)
  line L131 (108.9327, 27.0981) -> (104.6025, 29.5981)
  line L132 (8.0801, 38.3971) -> (3.75, 35.8971)
  line L133 (3.75, 35.8971) -> (3.75, 30.8971)
  line L134 (3.75, 30.8971) -> (8.0801, 28.3971)
  line L135 (8.0801, 28.3971) -> (12.4103, 30.8971)
  line L136 (12.4103, 30.8971) -> (12.4103, 35.8971)
  line L137 (12.4103, 35.8971) -> (8.0801, 38.3971)
  line L138 (18.2404, 38.3971) -> (13.9103, 35.8971)
  line L139 (13.9103, 35.8971) -> (13.9103, 30.8971)
  line L140 (13.9103, 30.8971) -> (18.2404, 28.3971)
  line L141 (18.2404, 28.3971) -> (22.5705, 30.8971)
  line L142 (22.5705, 30.8971) -> (22.5705, 35.8971)
  line L143 (22.5705, 35.8971) -> (18.2404, 38.3971)
  line L144 (28.4006, 38.3971) -> (24.0705, 35.8971)
  line L145 (24.0705, 35.8971) -> (24.0705, 30.8971)
  line L146 (24.0705, 30.8971) -> (28.4006, 28.3971)
  line L147 (28.4006, 28.3971) -> (32.7308, 30.8971)
  line L148 (32.7308, 30.8971) -> (32.7308, 35.8971)
  line L149 (32.7308, 35.8971) -> (28.4006, 38.3971)
  line L150 (38.5609, 38.3971) -> (34.2308, 35.8971)
  line L151 (34.2308, 35.8971) -> (34.2308, 30.8971)
  line L152 (34.2308, 30.8971) -> (38.5609, 28.3971)
  line L153 (38.5609, 28.3971) -> (42.891, 30.8971)
  line L154 (42.891, 30.8971) -> (42.891, 35.8971)
  line L155 (42.891, 35.8971) -> (38.5609, 38.3971)
  line L156 (48.7211, 38.3971) -> (44.391, 35.8971)
  line L157 (44.391, 35.8971) -> (44.391, 30.8971)
  line L158 (44.391, 30.8971) -> (48.7211, 28.3971)
  line L159 (48.7211, 28.3971) -> (53.0513, 30.8971)
  line L160 (53.0513, 30.8971) -> (53.0513, 35.8971)
  line L161 (53.0513, 35.8971) -> (48.7211, 38.3971)
  line L162 (58.8814, 38.3971) -> (54.5513, 35.8971)
  line L163 (54.5513, 35.8971) -> (54.5513, 30.8971)
  line L164 (54.5513, 30.8971) -> (58.8814, 28.3971)
  line L165 (58.8814, 28.3971) -> (63.2115, 30.8971)
  line L166 (63.2115, 30.8971) -> (63.2115, 35.8971)
  line L167 (63.2115, 35.8971) -> (58.8814, 38.3971)
  line L168 (69.0417, 38.3971) -> (64.7115, 35.8971)
  line L169 (64.7115, 35.8971) -> (64.7115, 30.8971)
  line L170 (64.7115, 30.8971) -> (69.0417, 28.3971)
  line L171 (69.0417, 28.3971) -> (73.3718, 30.8971)
  line L172 (73.3718, 30.8971) -> (73.3718, 35.8971)
  line L173 (73.3718, 35.8971) -> (69.0417, 38.3971)
  line L174 (79.2019, 38.3971) -> (74.8718, 35.8971)
  line L175 (74.8718, 35.8971) -> (74.8718, 30.8971)
  line L176 (74.8718, 30.8971) -> (79.2019, 28.3971)
  line L177 (79.2019, 28.3971) -> (83.532, 30.8971)
  line L178 (83.532, 30.8971) -> (83.532, 35.8971)
  line L179 (83.532, 35.8971) -> (79.2019, 38.3971)
  line L180 (89.3622, 38.3971) -> (85.032, 35.8971)
  line L181 (85.032, 35.8971) -> (85.032, 30.8971)
  line L182 (85.032, 30.8971) -> (89.3622, 28.3971)
  line L183 (89.3622, 28.3971) -> (93.6923, 30.8971)
  line L184 (93.6923, 30.8971) -> (93.6923, 35.8971)
  line L185 (93.6923, 35.8971) -> (89.3622, 38.3971)
  line L186 (99.5224, 38.3971) -> (95.1923, 35.8971)
  line L187 (95.1923, 35.8971) -> (95.1923, 30.8971)
  line L188 (95.1923, 30.8971) -> (99.5224, 28.3971)
  line L189 (99.5224, 28.3971) -> (103.8525, 30.8971)
  line L190 (103.8525, 30.8971) -> (103.8525, 35.8971)
  line L191 (103.8525, 35.8971) -> (99.5224, 38.3971)
  line L192 (3, 47.1962) -> (-1.3301, 44.6962)
  line L193 (-1.3301, 44.6962) -> (-1.3301, 39.6962)
  line L194 (-1.3301, 39.6962) -> (3, 37.1962)
  line L195 (3, 37.1962) -> (7.3301, 39.6962)
  line L196 (7.3301, 39.6962) -> (7.3301, 44.6962)
  line L197 (7.3301, 44.6962) -> (3, 47.1962)
  line L198 (13.1603, 47.1962) -> (8.8301, 44.6962)
  line L199 (8.8301, 44.6962) -> (8.8301, 39.6962)
  line L200 (8.8301, 39.6962) -> (13.1603, 37.1962)
  line L201 (13.1603, 37.1962) -> (17.4904, 39.6962)
  line L202 (17.4904, 39.6962) -> (17.4904, 44.6962)
  line L203 (17.4904, 44.6962) -> (13.1603, 47.1962)
  line L204 (23.3205, 47.1962) -> (18.9904, 44.6962)
  line L205 (18.9904, 44.6962) -> (18.9904, 39.6962)
  line L206 (18.9904, 39.6962) -> (23.3205, 37.1962)
  line L207 (23.3205, 37.1962) -> (27.6506, 39.6962)
  line L208 (27.6506, 39.6962) -> (27.6506, 44.6962)
  line L209 (27.6506, 44.6962) -> (23.3205, 47.1962)
  line L210 (33.4808, 47.1962) -> (29.1506, 44.6962)
  line L211 (29.1506, 44.6962) -> (29.1506, 39.6962)
  line L212 (29.1506, 39.6962) -> (33.4808, 37.1962)
  line L213 (33.4808, 37.1962) -> (37.8109, 39.6962)
  line L214 (37.8109, 39.6962) -> (37.8109, 44.6962)
  line L215 (37.8109, 44.6962) -> (33.4808, 47.1962)
  line L216 (43.641, 47.1962) -> (39.3109, 44.6962)
  line L217 (39.3109, 44.6962) -> (39.3109, 39.6962)
  line L218 (39.3109, 39.6962) -> (43.641, 37.1962)
  line L219 (43.641, 37.1962) -> (47.9711, 39.6962)
  line L220 (47.9711, 39.6962) -> (47.9711, 44.6962)
  line L221 (47.9711, 44.6962) -> (43.641, 47.1962)
  line L222 (53.8013, 47.1962) -> (49.4711, 44.6962)
  line L223 (49.4711, 44.6962) -> (49.4711, 39.6962)
  line L224 (49.4711, 39.6962) -> (53.8013, 37.1962)
  line L225 (53.8013, 37.1962) -> (58.1314, 39.6962)
  line L226 (58.1314, 39.6962) -> (58.1314, 44.6962)
  line L227 (58.1314, 44.6962) -> (53.8013, 47.1962)
  line L228 (63.9615, 47.1962) -> (59.6314, 44.6962)
  line L229 (59.6314, 44.6962) -> (59.6314, 39.6962)
  line L230 (59.6314, 39.6962) -> (63.9615, 37.1962)
  line L231 (63.9615, 37.1962) -> (68.2917, 39.6962)
  line L232 (68.2917, 39.6962) -> (68.2917, 44.6962)
  line L233 (68.2917, 44.6962) -> (63.9615, 47.1962)
  line L234 (74.1218, 47.1962) -> (69.7917, 44.6962)
  line L235 (69.7917, 44.6962) -> (69.7917, 39.6962)
  line L236 (69.7917, 39.6962) -> (74.1218, 37.1962)
  line L237 (74.1218, 37.1962) -> (78.4519, 39.6962)
  line L238 (78.4519, 39.6962) -> (78.4519, 44.6962)
  line L239 (78.4519, 44.6962) -> (74.1218, 47.1962)
  line L240 (84.282, 47.1962) -> (79.9519, 44.6962)
  line L241 (79.9519, 44.6962) -> (79.9519, 39.6962)
  line L242 (79.9519, 39.6962) -> (84.282, 37.1962)
  line L243 (84.282, 37.1962) -> (88.6122, 39.6962)
  line L244 (88.6122, 39.6962) -> (88.6122, 44.6962)
  line L245 (88.6122, 44.6962) -> (84.282, 47.1962)
  line L246 (94.4423, 47.1962) -> (90.1122, 44.6962)
  line L247 (90.1122, 44.6962) -> (90.1122, 39.6962)
  line L248 (90.1122, 39.6962) -> (94.4423, 37.1962)
  line L249 (94.4423, 37.1962) -> (98.7724, 39.6962)
  line L250 (98.7724, 39.6962) -> (98.7724, 44.6962)
  line L251 (98.7724, 44.6962) -> (94.4423, 47.1962)
  line L252 (104.6025, 47.1962) -> (100.2724, 44.6962)
  line L253 (100.2724, 44.6962) -> (100.2724, 39.6962)
  line L254 (100.2724, 39.6962) -> (104.6025, 37.1962)
  line L255 (104.6025, 37.1962) -> (108.9327, 39.6962)
  line L256 (108.9327, 39.6962) -> (108.9327, 44.6962)
  line L257 (108.9327, 44.6962) -> (104.6025, 47.1962)
  line L258 (8.0801, 55.9952) -> (3.75, 53.4952)
  line L259 (3.75, 53.4952) -> (3.75, 48.4952)
  line L260 (3.75, 48.4952) -> (8.0801, 45.9952)
  line L261 (8.0801, 45.9952) -> (12.4103, 48.4952)
  line L262 (12.4103, 48.4952) -> (12.4103, 53.4952)
  line L263 (12.4103, 53.4952) -> (8.0801, 55.9952)
  line L264 (18.2404, 55.9952) -> (13.9103, 53.4952)
  line L265 (13.9103, 53.4952) -> (13.9103, 48.4952)
  line L266 (13.9103, 48.4952) -> (18.2404, 45.9952)
  line L267 (18.2404, 45.9952) -> (22.5705, 48.4952)
  line L268 (22.5705, 48.4952) -> (22.5705, 53.4952)
  line L269 (22.5705, 53.4952) -> (18.2404, 55.9952)
  line L270 (28.4006, 55.9952) -> (24.0705, 53.4952)
  line L271 (24.0705, 53.4952) -> (24.0705, 48.4952)
  line L272 (24.0705, 48.4952) -> (28.4006, 45.9952)
  line L273 (28.4006, 45.9952) -> (32.7308, 48.4952)
  line L274 (32.7308, 48.4952) -> (32.7308, 53.4952)
  line L275 (32.7308, 53.4952) -> (28.4006, 55.9952)
  line L276 (38.5609, 55.9952) -> (34.2308, 53.4952)
  line L277 (34.2308, 53.4952) -> (34.2308, 48.4952)
  line L278 (34.2308, 48.4952) -> (38.5609, 45.9952)
  line L279 (38.5609, 45.9952) -> (42.891, 48.4952)
  line L280 (42.891, 48.4952) -> (42.891, 53.4952)
  line L281 (42.891, 53.4952) -> (38.5609, 55.9952)
  line L282 (48.7211, 55.9952) -> (44.391, 53.4952)
  line L283 (44.391, 53.4952) -> (44.391, 48.4952)
  line L284 (44.391, 48.4952) -> (48.7211, 45.9952)
  line L285 (48.7211, 45.9952) -> (53.0513, 48.4952)
  line L286 (53.0513, 48.4952) -> (53.0513, 53.4952)
  line L287 (53.0513, 53.4952) -> (48.7211, 55.9952)
  line L288 (58.8814, 55.9952) -> (54.5513, 53.4952)
  line L289 (54.5513, 53.4952) -> (54.5513, 48.4952)
  line L290 (54.5513, 48.4952) -> (58.8814, 45.9952)
  line L291 (58.8814, 45.9952) -> (63.2115, 48.4952)
  line L292 (63.2115, 48.4952) -> (63.2115, 53.4952)
  line L293 (63.2115, 53.4952) -> (58.8814, 55.9952)
  line L294 (69.0417, 55.9952) -> (64.7115, 53.4952)
  line L295 (64.7115, 53.4952) -> (64.7115, 48.4952)
  line L296 (64.7115, 48.4952) -> (69.0417, 45.9952)
  line L297 (69.0417, 45.9952) -> (73.3718, 48.4952)
  line L298 (73.3718, 48.4952) -> (73.3718, 53.4952)
  line L299 (73.3718, 53.4952) -> (69.0417, 55.9952)
  line L300 (79.2019, 55.9952) -> (74.8718, 53.4952)
  line L301 (74.8718, 53.4952) -> (74.8718, 48.4952)
  line L302 (74.8718, 48.4952) -> (79.2019, 45.9952)
  line L303 (79.2019, 45.9952) -> (83.532, 48.4952)
  line L304 (83.532, 48.4952) -> (83.532, 53.4952)
  line L305 (83.532, 53.4952) -> (79.2019, 55.9952)
  line L306 (89.3622, 55.9952) -> (85.032, 53.4952)
  line L307 (85.032, 53.4952) -> (85.032, 48.4952)
  line L308 (85.032, 48.4952) -> (89.3622, 45.9952)
  line L309 (89.3622, 45.9952) -> (93.6923, 48.4952)
  line L310 (93.6923, 48.4952) -> (93.6923, 53.4952)
  line L311 (93.6923, 53.4952) -> (89.3622, 55.9952)
  line L312 (99.5224, 55.9952) -> (95.1923, 53.4952)
  line L313 (95.1923, 53.4952) -> (95.1923, 48.4952)
  line L314 (95.1923, 48.4952) -> (99.5224, 45.9952)
  line L315 (99.5224, 45.9952) -> (103.8525, 48.4952)
  line L316 (103.8525, 48.4952) -> (103.8525, 53.4952)
  line L317 (103.8525, 53.4952) -> (99.5224, 55.9952)
  line L318 (3, 64.7942) -> (-1.3301, 62.2942)
  line L319 (-1.3301, 62.2942) -> (-1.3301, 57.2942)
  line L320 (-1.3301, 57.2942) -> (3, 54.7942)
  line L321 (3, 54.7942) -> (7.3301, 57.2942)
  line L322 (7.3301, 57.2942) -> (7.3301, 62.2942)
  line L323 (7.3301, 62.2942) -> (3, 64.7942)
  line L324 (13.1603, 64.7942) -> (8.8301, 62.2942)
  line L325 (8.8301, 62.2942) -> (8.8301, 57.2942)
  line L326 (8.8301, 57.2942) -> (13.1603, 54.7942)
  line L327 (13.1603, 54.7942) -> (17.4904, 57.2942)
  line L328 (17.4904, 57.2942) -> (17.4904, 62.2942)
  line L329 (17.4904, 62.2942) -> (13.1603, 64.7942)
  line L330 (23.3205, 64.7942) -> (18.9904, 62.2942)
  line L331 (18.9904, 62.2942) -> (18.9904, 57.2942)
  line L332 (18.9904, 57.2942) -> (23.3205, 54.7942)
  line L333 (23.3205, 54.7942) -> (27.6506, 57.2942)
  line L334 (27.6506, 57.2942) -> (27.6506, 62.2942)
  line L335 (27.6506, 62.2942) -> (23.3205, 64.7942)
  line L336 (33.4808, 64.7942) -> (29.1506, 62.2942)
  line L337 (29.1506, 62.2942) -> (29.1506, 57.2942)
  line L338 (29.1506, 57.2942) -> (33.4808, 54.7942)
  line L339 (33.4808, 54.7942) -> (37.8109, 57.2942)
  line L340 (37.8109, 57.2942) -> (37.8109, 62.2942)
  line L341 (37.8109, 62.2942) -> (33.4808, 64.7942)
  line L342 (43.641, 64.7942) -> (39.3109, 62.2942)
  line L343 (39.3109, 62.2942) -> (39.3109, 57.2942)
  line L344 (39.3109, 57.2942) -> (43.641, 54.7942)
  line L345 (43.641, 54.7942) -> (47.9711, 57.2942)
  line L346 (47.9711, 57.2942) -> (47.9711, 62.2942)
  line L347 (47.9711, 62.2942) -> (43.641, 64.7942)
  line L348 (53.8013, 64.7942) -> (49.4711, 62.2942)
  line L349 (49.4711, 62.2942) -> (49.4711, 57.2942)
  line L350 (49.4711, 57.2942) -> (53.8013, 54.7942)
  line L351 (53.8013, 54.7942) -> (58.1314, 57.2942)
  line L352 (58.1314, 57.2942) -> (58.1314, 62.2942)
  line L353 (58.1314, 62.2942) -> (53.8013, 64.7942)
  line L354 (63.9615, 64.7942) -> (59.6314, 62.2942)
  line L355 (59.6314, 62.2942) -> (59.6314, 57.2942)
  line L356 (59.6314, 57.2942) -> (63.9615, 54.7942)
  line L357 (63.9615, 54.7942) -> (68.2917, 57.2942)
  line L358 (68.2917, 57.2942) -> (68.2917, 62.2942)
  line L359 (68.2917, 62.2942) -> (63.9615, 64.7942)
  line L360 (74.1218, 64.7942) -> (69.7917, 62.2942)
  line L361 (69.7917, 62.2942) -> (69.7917, 57.2942)
  line L362 (69.7917, 57.2942) -> (74.1218, 54.7942)
  line L363 (74.1218, 54.7942) -> (78.4519, 57.2942)
  line L364 (78.4519, 57.2942) -> (78.4519, 62.2942)
  line L365 (78.4519, 62.2942) -> (74.1218, 64.7942)
  line L366 (84.282, 64.7942) -> (79.9519, 62.2942)
  line L367 (79.9519, 62.2942) -> (79.9519, 57.2942)
  line L368 (79.9519, 57.2942) -> (84.282, 54.7942)
  line L369 (84.282, 54.7942) -> (88.6122, 57.2942)
  line L370 (88.6122, 57.2942) -> (88.6122, 62.2942)
  line L371 (88.6122, 62.2942) -> (84.282, 64.7942)
  line L372 (94.4423, 64.7942) -> (90.1122, 62.2942)
  line L373 (90.1122, 62.2942) -> (90.1122, 57.2942)
  line L374 (90.1122, 57.2942) -> (94.4423, 54.7942)
  line L375 (94.4423, 54.7942) -> (98.7724, 57.2942)
  line L376 (98.7724, 57.2942) -> (98.7724, 62.2942)
  line L377 (98.7724, 62.2942) -> (94.4423, 64.7942)
  line L378 (104.6025, 64.7942) -> (100.2724, 62.2942)
  line L379 (100.2724, 62.2942) -> (100.2724, 57.2942)
  line L380 (100.2724, 57.2942) -> (104.6025, 54.7942)
  line L381 (104.6025, 54.7942) -> (108.9327, 57.2942)
  line L382 (108.9327, 57.2942) -> (108.9327, 62.2942)
  line L383 (108.9327, 62.2942) -> (104.6025, 64.7942)
  line L384 (8.0801, 73.5933) -> (3.75, 71.0933)
  line L385 (3.75, 71.0933) -> (3.75, 66.0933)
  line L386 (3.75, 66.0933) -> (8.0801, 63.5933)
  line L387 (8.0801, 63.5933) -> (12.4103, 66.0933)
  line L388 (12.4103, 66.0933) -> (12.4103, 71.0933)
  line L389 (12.4103, 71.0933) -> (8.0801, 73.5933)
  line L390 (18.2404, 73.5933) -> (13.9103, 71.0933)
  line L391 (13.9103, 71.0933) -> (13.9103, 66.0933)
  line L392 (13.9103, 66.0933) -> (18.2404, 63.5933)
  line L393 (18.2404, 63.5933) -> (22.5705, 66.0933)
  line L394 (22.5705, 66.0933) -> (22.5705, 71.0933)
  line L395 (22.5705, 71.0933) -> (18.2404, 73.5933)
  line L396 (28.4006, 73.5933) -> (24.0705, 71.0933)
  line L397 (24.0705, 71.0933) -> (24.0705, 66.0933)
  line L398 (24.0705, 66.0933) -> (28.4006, 63.5933)
  line L399 (28.4006, 63.5933) -> (32.7308, 66.0933)
  line L400 (32.7308, 66.0933) -> (32.7308, 71.0933)
  line L401 (32.7308, 71.0933) -> (28.4006, 73.5933)
  line L402 (38.5609, 73.5933) -> (34.2308, 71.0933)
  line L403 (34.2308, 71.0933) -> (34.2308, 66.0933)
  line L404 (34.2308, 66.0933) -> (38.5609, 63.5933)
  line L405 (38.5609, 63.5933) -> (42.891, 66.0933)
  line L406 (42.891, 66.0933) -> (42.891, 71.0933)
  line L407 (42.891, 71.0933) -> (38.5609, 73.5933)
  line L408 (48.7211, 73.5933) -> (44.391, 71.0933)
  line L409 (44.391, 71.0933) -> (44.391, 66.0933)
  line L410 (44.391, 66.0933) -> (48.7211, 63.5933)
  line L411 (48.7211, 63.5933) -> (53.0513, 66.0933)
  line L412 (53.0513, 66.0933) -> (53.0513, 71.0933)
  line L413 (53.0513, 71.0933) -> (48.7211, 73.5933)
  line L414 (58.8814, 73.5933) -> (54.5513, 71.0933)
  line L415 (54.5513, 71.0933) -> (54.5513, 66.0933)
  line L416 (54.5513, 66.0933) -> (58.8814, 63.5933)
  line L417 (58.8814, 63.5933) -> (63.2115, 66.0933)
  line L418 (63.2115, 66.0933) -> (63.2115, 71.0933)
  line L419 (63.2115, 71.0933) -> (58.8814, 73.5933)
  line L420 (69.0417, 73.5933) -> (64.7115, 71.0933)
  line L421 (64.7115, 71.0933) -> (64.7115, 66.0933)
  line L422 (64.7115, 66.0933) -> (69.0417, 63.5933)
  line L423 (69.0417, 63.5933) -> (73.3718, 66.0933)
  line L424 (73.3718, 66.0933) -> (73.3718, 71.0933)
  line L425 (73.3718, 71.0933) -> (69.0417, 73.5933)
  line L426 (79.2019, 73.5933) -> (74.8718, 71.0933)
  line L427 (74.8718, 71.0933) -> (74.8718, 66.0933)
  line L428 (74.8718, 66.0933) -> (79.2019, 63.5933)
  line L429 (79.2019, 63.5933) -> (83.532, 66.0933)
  line L430 (83.532, 66.0933) -> (83.532, 71.0933)
  line L431 (83.532, 71.0933) -> (79.2019, 73.5933)
  line L432 (89.3622, 73.5933) -> (85.032, 71.0933)
  line L433 (85.032, 71.0933) -> (85.032, 66.0933)
  line L434 (85.032, 66.0933) -> (89.3622, 63.5933)
  line L435 (89.3622, 63.5933) -> (93.6923, 66.0933)
  line L436 (93.6923, 66.0933) -> (93.6923, 71.0933)
  line L437 (93.6923, 71.0933) -> (89.3622, 73.5933)
  line L438 (99.5224, 73.5933) -> (95.1923, 71.0933)
  line L439 (95.1923, 71.0933) -> (95.1923, 66.0933)
  line L440 (95.1923, 66.0933) -> (99.5224, 63.5933)
  line L441 (99.5224, 63.5933) -> (103.8525, 66.0933)
  line L442 (103.8525, 66.0933) -> (103.8525, 71.0933)
  line L443 (103.8525, 71.0933) -> (99.5224, 73.5933)
  line L444 (3, 82.3923) -> (-1.3301, 79.8923)
  line L445 (-1.3301, 79.8923) -> (-1.3301, 74.8923)
  line L446 (-1.3301, 74.8923) -> (3, 72.3923)
  line L447 (3, 72.3923) -> (7.3301, 74.8923)
  line L448 (7.3301, 74.8923) -> (7.3301, 79.8923)
  line L449 (7.3301, 79.8923) -> (3, 82.3923)
  line L450 (13.1603, 82.3923) -> (8.8301, 79.8923)
  line L451 (8.8301, 79.8923) -> (8.8301, 74.8923)
  line L452 (8.8301, 74.8923) -> (13.1603, 72.3923)
  line L453 (13.1603, 72.3923) -> (17.4904, 74.8923)
  line L454 (17.4904, 74.8923) -> (17.4904, 79.8923)
  line L455 (17.4904, 79.8923) -> (13.1603, 82.3923)
  line L456 (23.3205, 82.3923) -> (18.9904, 79.8923)
  line L457 (18.9904, 79.8923) -> (18.9904, 74.8923)
  line L458 (18.9904, 74.8923) -> (23.3205, 72.3923)
  line L459 (23.3205, 72.3923) -> (27.6506, 74.8923)
  line L460 (27.6506, 74.8923) -> (27.6506, 79.8923)
  line L461 (27.6506, 79.8923) -> (23.3205, 82.3923)
  line L462 (33.4808, 82.3923) -> (29.1506, 79.8923)
  line L463 (29.1506, 79.8923) -> (29.1506, 74.8923)
  line L464 (29.1506, 74.8923) -> (33.4808, 72.3923)
  line L465 (33.4808, 72.3923) -> (37.8109, 74.8923)
  line L466 (37.8109, 74.8923) -> (37.8109, 79.8923)
  line L467 (37.8109, 79.8923) -> (33.4808, 82.3923)
  line L468 (43.641, 82.3923) -> (39.3109, 79.8923)
  line L469 (39.3109, 79.8923) -> (39.3109, 74.8923)